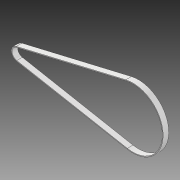
# Autodesk Inventor part: Rubberband
Saved by Autodesk Inventor 2020 (Build 240168000, 168)
## iProperties
Created: 2021-05-16
Part Number: Rubberband
Material: Generic
Document SubType Name: Modeling
Designer: DDeGo
Density: 1 g/cm^3
Appearance: Default
Author: DDeGo
Autodesk Inventor part; units mm, degrees
ref_plane "YZ Plane" through (0, 0, 0) normal (1, 0, 0) x (0, 1, 0)
ref_plane "XZ Plane" through (0, 0, 0) normal (0, 1, 0) x (-1, 0, 0)
ref_plane "XY Plane" through (0, 0, 0) normal (0, 0, 1) x (1, 0, 0)
sketch "Sketch1" plane through (0, 0, 0) normal (0, 0, 1) x (1, 0, 0)
  arc A0 (-0.8035, 3.4065) -> (-0.6457, -3.4399) centre (0, 0) ccw
  arc A1 (66.6791, -16.0777) -> (65.8677, 19.1325) centre (70, 1.6133) ccw
  line L0 (-0.8035, 3.4065) -> (65.8677, 19.1325)
  line L1 (66.6791, -16.0777) -> (-0.6457, -3.4399)
  line L2 (0, 0) -> (70, 1.6133) construction
  line L3 (65.7529, 19.6192) -> (-0.9183, 3.8932)
  arc A2 (-0.9183, 3.8932) -> (-0.738, -3.9313) centre (0, 0) ccw
  line L4 (-0.738, -3.9313) -> (66.5869, -16.5692)
  arc A3 (66.5869, -16.5692) -> (65.7529, 19.6192) centre (70, 1.6133) ccw
  circle A4 centre (0, 0) radius 3.5 construction
  circle A5 centre (70, 1.6133) radius 18 construction
  dimension "d0" = 0.5
  constraints: 10 end point, 8 point on circle, 4 centre point, 4 tangent, 2 coincident, 2 concentric, 3 other
  measures "d0" distance between parallel lines of L0 L3
extrude "Extrusion1" add sketch "Sketch1" along normal blind 3.4
body "Solid1"
